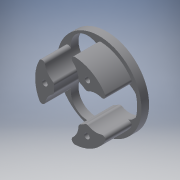
# Autodesk Inventor part: LayerBase2
Saved by Autodesk Inventor 2019 (Build 230136000, 136)
## iProperties
Created: 2022-08-24
Part Number: LayerBase2
Material: Generic
Document SubType Name: Modeling
Designer: zreik
Density: 1 g/cm^3
Appearance: Default
Author: zreik
Autodesk Inventor part; units mm, degrees
ref_plane "YZ Plane" through (0, 0, 0) normal (1, 0, 0) x (0, 1, 0)
ref_plane "XZ Plane" through (0, 0, 0) normal (0, 1, 0) x (-1, 0, 0)
ref_plane "XY Plane" through (0, 0, 0) normal (0, 0, 1) x (1, 0, 0)
sketch "Sketch1" plane through (0, 0, 0) normal (0, 0, 1) x (1, 0, 0)
  circle A0 centre (0, 0) radius 24.75
  circle A1 centre (0, 0) radius 12.5
  dimension "d0" = 49.5
  dimension "d1" = 25
  constraints: 2 centre point, 2 coincident
  measures "d0" diameter of A0
  measures "d1" diameter of A1
extrude "Extrusion1" add sketch "Sketch1" along normal blind 22
sketch "Sketch2" plane through (0, 0, 22) normal (0, 0, 1) x (1, 0, 0)
  circle A0 centre (15, 0) radius 11
  point P0 (0, 0)
  dimension "d4" = 15
  dimension "d5" = 0
  dimension "d6" = 22
  constraints: 1 centre point
  measures "d4" distance of point (0, 0) A0.centre
  measures "d5" vertical distance of point (0, 0) A0.centre
  measures "d6" diameter of A0
extrude "Extrusion2" cut sketch "Sketch2" against normal blind 22
sketch "Sketch3" plane through (0, 0, 0) normal (0, 0, -1) x (-1, 0, 0)
  circle A0 centre (0, 0) radius 24.75
  circle A1 centre (0, 0) radius 27.5
  dimension "d13" = 49.5
  dimension "d14" = 55
  constraints: 2 centre point, 2 coincident
  measures "d13" diameter of A0
  measures "d14" diameter of A1
extrude "Extrusion3" add sketch "Sketch3" against normal blind 5
fillet "Fillet1" radius 2 4 edges at (8.675, 8.9997, 11) (8.675, -8.9997, 11) (23.8854, 6.4845, 13.5) (23.8854, -6.4845, 13.5)
pattern_circular "Circular Pattern1" count 3 over 360 about axis through (0, 0, 0) along (0, 0, 1) of "Extrusion2", "Fillet1"
sketch "Sketch4" plane through (0, 0, 22) normal (0, 0, 1) x (1, 0, 0)
  circle A0 centre (9, -16) radius 1.75
  point P0 (0, 0)
  dimension "d17" = 3.5
  dimension "d18" = 16
  dimension "d19" = 9
  constraints: 1 centre point
  measures "d17" diameter of A0
  measures "d18" vertical distance of point (0, 0) A0.centre
  measures "d19" horizontal distance of point (0, 0) A0.centre
extrude "Extrusion4" cut sketch "Sketch4" against normal through all
pattern_circular "Circular Pattern2" count 3 over 360 about axis through (0, 0, 0) along (0, 0, 1) of "Extrusion4"
body "Solid1"
